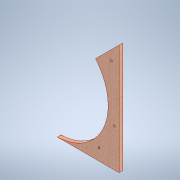
# Autodesk Inventor part: Hood
Saved by Autodesk Inventor 2020 (Build 240168000, 168)
## iProperties
Created: 2020-01-13
Part Number: Hood
Material: Wood (Oak)
Document SubType Name: Modeling
Designer: autum
Density: 0.76 g/cm^3
Appearance: White Oak - Natural Medium Gloss
Author: autum
Autodesk Inventor part; units mm, degrees
ref_plane "YZ Plane" through (0, 0, 0) normal (1, 0, 0) x (0, 1, 0)
ref_plane "XZ Plane" through (0, 0, 0) normal (0, 1, 0) x (-1, 0, 0)
ref_plane "XY Plane" through (0, 0, 0) normal (0, 0, 1) x (1, 0, 0)
sketch "Sketch1" plane through (0, 0, 0) normal (0, 0, 1) x (1, 0, 0)
  arc A0 (295.1408, -159.2152) -> (331.6912, 112.9068) centre (191.7703, -6.8152) ccw
  line L0 (414.0203, 195.2359) -> (414.0203, -190.9652)
  line L1 (414.0203, -190.9652) -> (198.1203, -190.9652)
  arc A1 (198.1203, -190.8557) -> (331.6912, 112.9068) centre (191.7703, -6.8152) ccw
  arc A2 (198.1203, -190.8557) -> (331.6912, 112.9068) centre (191.7703, -6.8152) ccw
  line L2 (414.0203, 195.2359) -> (501.2785, 195.2359) construction
  line L3 (414.0203, 195.2359) -> (331.6912, 112.9068)
  line L4 (414.0203, 195.2359) -> (530.4512, 195.2359) construction
  line L5 (198.1203, -190.8557) -> (198.1203, -190.9652)
  point P0 (347.2273, 121.372)
  point P1 (295.1408, -159.2152)
  dimension "d5" = 184.15
  dimension "d10" = 135
  dimension "d14" = 222.25
  dimension "d17" = 119.722
  constraints: 12 end point, 6 point on circle, 3 centre point, 2 coincident, 2 horizontal, 2 vertical, 1 equal length, 1 perpendicular
  measures "d5" radius of A0
  measures "d10" angle of L3 L4
  measures "d14" distance from line of L0 A0.centre
  measures "d17" vertical distance of L3.end A0.centre
extrude "Extrusion2" add sketch "Sketch1" along normal blind 12.7
sketch "Sketch2" plane through (0, 0, 0) normal (0, 0, -1) x (-1, 0, 0)
  line L0 (-414.0203, -190.9652) -> (-414.0203, 195.2359) projected
  line L1 (-198.1203, -190.9652) -> (-414.0203, -190.9652) projected
  point P0 (0, 0)
  point P1 (-344.1703, -150.3252)
  point P2 (-397.5103, -57.6152)
  point P3 (-387.3503, 134.1548)
  dimension "d18" = 69.85
  dimension "d19" = 40.64
  dimension "d20" = 133.35
  dimension "d21" = 16.51
  dimension "d22" = 325.12
  dimension "d23" = 26.67
  measures "d18" distance from line of point (-344.17, -150.325) L0
  measures "d19" vertical distance of L0.start point (-344.17, -150.325)
  measures "d20" vertical distance of L0.start point (-397.51, -57.615)
  measures "d21" distance from line of L0 point (-397.51, -57.615)
  measures "d22" distance from line of L1 point (-387.35, 134.155)
  measures "d23" distance from line of L0 point (-387.35, 134.155)
hole "Hole1" at (344.1703, -150.3252, 0) at (397.5103, -57.6152, 0) at (387.3503, 134.1548, 0) direction (0, 0, 1) diameter 6.7564 end through all
body "Solid2"
